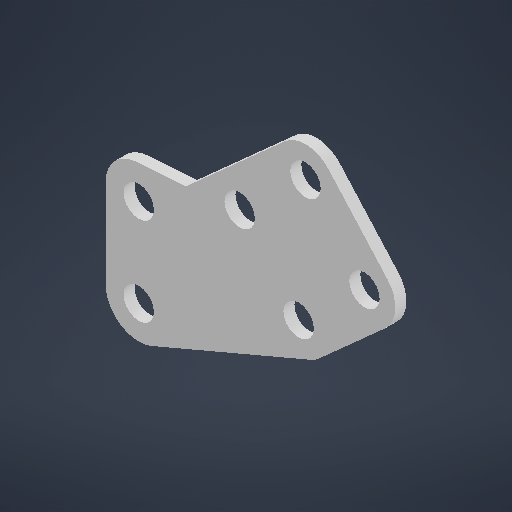
# Autodesk Inventor part: lbMountInside
Saved by Autodesk Inventor 2025.2 (Build 292293000, 293)
## iProperties
Created: 2025-03-26
Part Number: lbMountInside
Material: Generic
Document SubType Name: Modeling
Designer: roejo
Density: 1 g/cm^3
Appearance: Default
Author: roejo
Autodesk Inventor part; units mm, degrees
ref_plane "YZ Plane" through (0, 0, 0) normal (1, 0, 0) x (0, 1, 0)
ref_plane "XZ Plane" through (0, 0, 0) normal (0, 1, 0) x (-1, 0, 0)
ref_plane "XY Plane" through (0, 0, 0) normal (0, 0, 1) x (1, 0, 0)
sketch "Sketch1" plane through (0, 0, 0) normal (0, 0, 1) x (1, 0, 0)
  circle A0 centre (-14.5571, -13.0053) radius 2.1844
  circle A1 centre (-14.5571, -0.3053) radius 2.1844
  circle A2 centre (9.4013, 14.3429) radius 2.1844
  circle A3 centre (17.8732, 4.8815) radius 2.1844
  circle A4 centre (8.4118, -3.5903) radius 2.1844
  circle A5 centre (-0.06, 5.871) radius 2.1844
  circle A6 centre (9.4013, 14.3429) radius 4.445
  circle A7 centre (17.8732, 4.8815) radius 4.445
  circle A8 centre (8.4118, -3.5903) radius 4.445
  circle A9 centre (-14.5571, -0.3053) radius 4.7625
  circle A10 centre (-14.5571, -13.0053) radius 4.7625
  circle A11 centre (-0.06, 5.871) radius 4.445
  line L0 (-0.06, 5.871) -> (8.4118, -3.5903)
  line L1 (8.4118, -3.5903) -> (11.377, -6.9018)
  line L2 (-19.3196, -0.3053) -> (-19.3196, -13.0053)
  line L3 (11.377, -6.9018) -> (20.8482, 1.5789)
  line L4 (10.1502, -7.6813) -> (-12.6946, -17.3885)
  line L5 (21.1847, 7.8467) -> (12.7128, 17.3081)
  line L6 (6.4362, 17.6544) -> (-3.0252, 9.1825)
  line L7 (-3.0252, 9.1825) -> (-7.7559, 4.9466)
  line L8 (-7.7559, 4.9466) -> (-14.8907, 4.4455)
  point P0 (0, 0)
  dimension "d5" = 8.89
  dimension "d0" = 8.89
  dimension "d1" = 8.89
  dimension "d2" = 8.89
  dimension "d3" = 9.525
  dimension "d4" = 9.525
  dimension "d9" = 6.35
  constraints: 18 end point, 11 centre point, 11 point on circle, 6 coincident, 6 tangent, 2 point on line, 4 other
  measures "d0" diameter of A6
  measures "d1" diameter of A7
  measures "d2" diameter of A8
  measures "d3" diameter of A9
  measures "d4" diameter of A10
  measures "d9" distance of L6.end L7.end
extrude "Extrusion1" add sketch "Sketch1" along normal blind 1.5875 contours A4 L0 A8 L1 | A4 L1 A8 L0 | A7 | L0 A11 L6 A6 L5 A7 L3 A8 | A8 L4 A10 L2 A9 L8 L7 A11 L0 | A11 | A10 | A6 | A9
body "Solid1"
